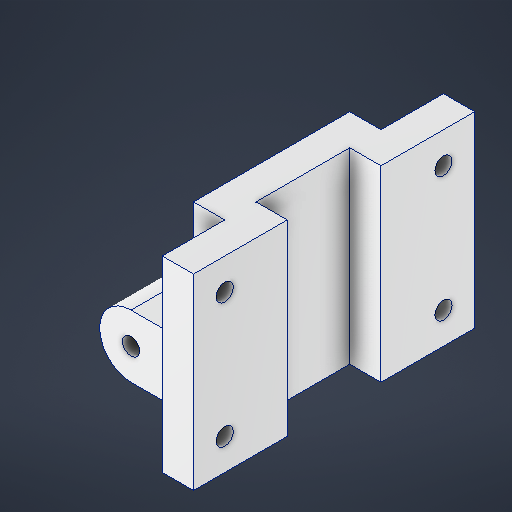
# Autodesk Inventor part: MMAE 232 Assignment 1d-Nicholas Skiba
Saved by Autodesk Inventor 2026.1 (Build 301233000, 233)
## iProperties
Created: 2025-08-25
Part Number: MMAE 232 Assignment 1d-Nicholas Skiba
Material: Aluminum 6061
Document SubType Name: Modeling
Designer: Nick
Density: 2.7 g/cm^3
Appearance: Aluminum - Flat
Mass: 255.348 g
Surface Area: 229.017 cm^2
Volume: 94.5733 cm^3
Author: Nick
Autodesk Inventor part; units mm, degrees
ref_plane "YZ Plane" through (0, 0, 0) normal (1, 0, 0) x (0, 1, 0)
ref_plane "XZ Plane" through (0, 0, 0) normal (0, 1, 0) x (-1, 0, 0)
sketch "Sketch1" plane through (0, 0, 0) normal (0, 1, 0) x (-1, 0, 0)
  line L0 (0, 0) -> (10, 0)
  line L1 (0, 0) -> (0, -30)
  line L2 (0, -30) -> (10, -30)
  line L3 (10, -30) -> (10, -60)
  line L4 (10, -60) -> (0, -60)
  line L5 (0, -60) -> (0, -90)
  line L6 (0, -90) -> (10, -90)
  line L7 (10, -90) -> (10, -70)
  line L8 (10, -70) -> (20, -70)
  line L9 (20, -70) -> (20, -20)
  line L10 (20, -20) -> (10, -20)
  line L11 (10, -20) -> (10, 0)
  dimension "d0" = 10
  dimension "d1" = 30
  dimension "d2" = 10
  dimension "d3" = 30
  dimension "d4" = 10
  dimension "d5" = 30
  dimension "d6" = 10
  dimension "d7" = 20
  dimension "d8" = 10
  dimension "d9" = 50
  constraints: 24 end point, 5 perpendicular, 5 point on line, 1 horizontal, 1 vertical
  measures "d0" distance of L0.start L0.end
  measures "d1" distance of L0.start L1.end
  measures "d2" distance of L1.end L2.end
  measures "d3" distance of L2.end L3.end
  measures "d4" distance of L3.end L4.end
  measures "d5" distance of L4.end L5.end
  measures "d6" distance of L5.end L6.end
  measures "d7" distance of L6.end L7.end
  measures "d8" distance of L7.end L8.end
  measures "d9" distance of L8.end L9.end
extrude "Extrusion1" add sketch "Sketch1" along normal blind 60
sketch "Sketch2" plane through (-10, 0, -90) normal (-1, 0, 0) x (0, 0, 1)
  line L0 (30, 60) -> (0, 60) projected
  line L1 (0, 60) -> (0, 32)
  line L2 (0, 0) -> (0, 60) projected
  line L3 (0, 32) -> (20, 32)
  line L4 (20, 32) -> (20, 28)
  line L5 (20, 28) -> (0, 28)
  line L6 (0, 28) -> (0, 32)
  line L7 (60, 60) -> (30, 60) projected
  line L8 (45, 60) -> (45, 0)
  line L9 (60, 0) -> (30, 0) projected
  line L10 (90, 0) -> (90, 60)
  line L11 (90, 32) -> (70, 32)
  line L12 (70, 32) -> (70, 28)
  line L13 (70, 28) -> (90, 28)
  line L14 (90, 28) -> (90, 32)
  dimension "d12" = 28
  dimension "d13" = 20
  dimension "d14" = 4
  constraints: 22 end point, 6 symmetric about line, 2 midpoint, 2 parallel, 2 point on line, 1 horizontal, 1 perpendicular
  measures "d12" distance of L0.end L1.end
  measures "d13" distance of L4.end L5.end
  measures "d14" distance of L3.end L4.end
extrude "Extrusion2" add sketch "Sketch2" along normal blind 10
sketch "Sketch3" plane through (-10, 32, -70) normal (0, 1, 0) x (1, 0, 0)
  line L0 (-10, 0) -> (-10, -50) projected
  line L1 (10, 20) -> (0, 20) projected
  line L2 (-10, 0) -> (0, 20)
  line L3 (0, 20) -> (-10, 20)
  line L4 (-10, 0) -> (-10, 20) projected
  line L5 (-10, 20) -> (-10, 0)
  line L6 (-10, -50) -> (0, -50) projected
  line L7 (0, -70) -> (10, -70) projected
  line L8 (-10, -50) -> (0, -70)
  line L9 (0, -70) -> (-10, -70)
  line L10 (-10, -70) -> (-10, -50)
  constraints: 12 end point, 3 collinear
extrude "Extrusion3" cut sketch "Sketch3" against normal blind 10
sketch "Sketch4" plane through (-10, 0, -70) normal (0, 0, -1) x (-1, 0, 0)
  line L0 (0, 32) -> (0, 60) projected
  line L1 (0, 60) -> (0, 10)
  line L2 (0, 10) -> (30, 10) construction
  circle A0 centre (30, 10) radius 2.75
  arc A1 (30, 0) -> (30, 20) centre (30, 10) ccw
  line L3 (10, 0) -> (0, 0) projected
  line L4 (0, 0) -> (30, 0)
  line L5 (0, 0) -> (0, 28) projected
  line L6 (0, 0) -> (0, 20)
  line L7 (0, 20) -> (30, 20)
  line L8 (10, 0) -> (10, 28) projected
  line L9 (10, 20) -> (10, 0)
  point P0 (-10, 0)
  dimension "d19" = 50
  dimension "d20" = 30
  dimension "d21" = 5.5
  dimension "d22" = 20
  constraints: 12 end point, 2 centre point, 2 coincident, 2 collinear, 2 perpendicular, 2 point on circle, 2 point on line, 2 tangent
  measures "d19" distance of L0.end L1.end
  measures "d20" distance of L1.end L2.end
  measures "d21" diameter of A0
  measures "d22" diameter of A1
extrude "Extrusion4" add sketch "Sketch4" against normal blind 50 contours L7 A1 L4 L8
ref_plane "Work Plane1" through (-20, 20, -47) normal (0, 0, -1) x (-1, 0, 0)
sketch "Sketch6" plane through (-20, 20, -47) normal (0, 0, -1) x (-1, 0, 0)
  line L0 (0, 40) -> (-10, 40) projected
  line L1 (0, 40) -> (28.4336, -4.6265)
  arc A0 (20, -20) -> (20, 0) centre (20, -10) ccw projected
  arc A1 (20, -20) -> (20, 0) centre (20, -10) ccw projected
  line L2 (28.4336, -4.6265) -> (-1.843, -4.6265)
  line L3 (-20, -20) -> (-20, 40) projected
  line L4 (-1.843, -4.6265) -> (-1.843, 40)
  constraints: 6 end point, 2 perpendicular, 1 point on circle, 1 point on line, 1 tangent
extrude "Extrusion6" add sketch "Sketch6" against normal blind 4
sketch "Sketch7" plane through (-10, 60, -90) normal (-1, 0, 0) x (0, 0, 1)
  line L0 (90, -28) -> (90, 0) projected
  line L1 (70, 0) -> (90, 0) projected
  line L2 (70, -60) -> (90, -60) projected
  line L3 (90, -60) -> (90, -32) projected
  line L4 (0, -60) -> (0, -32) projected
  line L5 (0, -60) -> (20, -60) projected
  line L6 (0, -28) -> (0, 0) projected
  line L7 (0, 0) -> (20, 0) projected
  point P0 (10, -10)
  point P1 (10, -50)
  point P2 (80, -50)
  point P3 (80, -10)
  dimension "d39" = 10
  dimension "d40" = 10
  dimension "d41" = 10
  dimension "d42" = 10
  dimension "d43" = 10
  dimension "d44" = 10
  dimension "d45" = 10
  dimension "d46" = 10
  measures "d39" distance from line of L0 point (80, -10)
  measures "d40" distance from line of L1 point (80, -10)
  measures "d41" distance from line of L2 point (80, -50)
  measures "d42" distance from line of L3 point (80, -50)
  measures "d43" distance from line of L4 point (10, -50)
  measures "d44" distance from line of L5 point (10, -50)
  measures "d45" distance from line of L6 point (10, -10)
  measures "d46" distance from line of L7 point (10, -10)
hole "Hole1" at (-10, 50, -80) at (-10, 10, -80) at (-10, 10, -10) at (-10, 50, -10) direction (1, 0, 0) diameter 5.5 end through all
body "Solid1"
